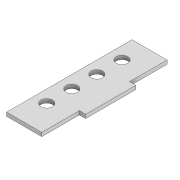
# Autodesk Inventor part: Lateral BNC
Saved by Autodesk Inventor 2020 (Build 240168000, 168)
## iProperties
Created: 2020-11-07
Part Number: Lateral BNC
Material: Generic
Document SubType Name: Modeling
Designer: ferrerx
Density: 1 g/cm^3
Appearance: Default
Author: ferrerx
Autodesk Inventor part; units mm, degrees
ref_plane "YZ Plane" through (0, 0, 0) normal (1, 0, 0) x (0, 1, 0)
ref_plane "XZ Plane" through (0, 0, 0) normal (0, 1, 0) x (-1, 0, 0)
ref_plane "XY Plane" through (0, 0, 0) normal (0, 0, 1) x (1, 0, 0)
sketch "Sketch1" plane through (0, 0, 0) normal (0, 1, 0) x (-1, 0, 0)
  line L0 (0, 0) -> (28, 0)
  line L1 (28, 0) -> (28, -100)
  line L2 (28, -100) -> (0, -100)
  line L3 (0, -100) -> (0, 0)
  line L4 (0, -30) -> (-5, -30)
  line L5 (-5, -30) -> (-5, -70)
  line L6 (-5, -70) -> (0, -70)
  line L7 (0, -70) -> (0, -30)
  line L8 (28, -50) -> (0, -50) construction
  line L9 (-5, -50) -> (0, -50) construction
  point P0 (0, -70)
  dimension "d0" = 100
  dimension "d1" = 5
  dimension "d2" = 40
  dimension "d3" = 28
  constraints: 20 end point, 4 midpoint, 4 parallel, 2 horizontal, 2 perpendicular, 1 collinear, 1 point on line
  measures "d0" distance of L2.end L0.start
  measures "d1" distance of L5.end L6.end
  measures "d2" distance of L4.end L5.end
  measures "d3" distance of L1.end L2.end
extrude "Extrusion1" add sketch "Sketch1" along normal blind 3
sketch "Sketch2" plane through (0, 3, 0) normal (0, 1, 0) x (1, 0, 0)
  line L0 (-28, 0) -> (0, 0) projected
  line L1 (-18, 0) -> (-18, 81.6583) construction
  circle A0 centre (-18, 22) radius 4.6
  line L2 (0, 0) -> (0, 30) projected
  circle A1 centre (-18, 42) radius 4.6
  circle A2 centre (-18, 62) radius 4.6
  circle A3 centre (-18, 82) radius 4.6
  dimension "d6" = 9.2
  dimension "d7" = 18
  dimension "d8" = 22
  dimension "d11" = 20
  constraints: 4 centre point, 2 end point, 2 point on line, 2 vertical, 6 other
  measures "d6" diameter of A0
  measures "d7" distance from line of L2 A0.centre
  measures "d8" distance from line of L0 A0.centre
  measures "d11" distance of A0.centre A1.centre
extrude "Extrusion2" cut sketch "Sketch2" against normal blind 5
body "Solid1"
